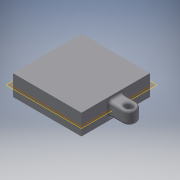
# Autodesk Inventor part: Casing_Part3
Saved by Autodesk Inventor 2019 (Build 230136000, 136)
## iProperties
Created: 2020-12-20
Part Number: Casing_Part3
Material: Generic
Document SubType Name: Modeling
Designer: nicolas
Density: 1 g/cm^3
Appearance: Default
Author: nicolas
Autodesk Inventor part; units mm, degrees
ref_plane "YZ Plane" through (0, 0, 0) normal (1, 0, 0) x (0, 1, 0)
ref_plane "XZ Plane" through (0, 0, 0) normal (0, 1, 0) x (-1, 0, 0)
ref_plane "XY Plane" through (0, 0, 0) normal (0, 0, 1) x (1, 0, 0)
sketch "Sketch1" plane through (0, 0, 0) normal (0, 1, 0) x (-1, 0, 0)
  line L0 (0, 0) -> (-50, 0)
  line L1 (-50, 0) -> (-50, -50)
  line L2 (-50, -50) -> (0, -50)
  line L3 (0, -50) -> (0, 0)
  dimension "d0" = 50
  dimension "d1" = 50
  constraints: 8 end point, 2 parallel, 1 horizontal, 1 perpendicular
  measures "d0" distance of L2.end L1.end
  measures "d1" distance of L1.end L0.end
extrude "Extrusion1" add sketch "Sketch1" along normal blind 15
ref_plane "Work Plane1" through (0, 7.5, 0) normal (0, 1, 0) x (1, 0, 0)
sketch "Sketch2" plane through (0, 7.5, 0) normal (0, 1, 0) x (1, 0, 0)
  line L0 (50, 20) -> (60, 20)
  line L1 (60, 20) -> (60, 30) construction
  line L2 (60, 30) -> (50, 30)
  line L3 (50, 30) -> (50, 20)
  line L4 (50, 20) -> (60, 30) construction
  line L5 (60, 20) -> (50, 30) construction
  line L6 (50, 0) -> (50, 50) projected
  arc A0 (60, 20) -> (60, 30) centre (60, 25) ccw
  line L7 (50, 25) -> (60, 25) construction
  point P0 (0, 0)
  dimension "d4" = 10
  dimension "d5" = 10
  constraints: 14 end point, 3 midpoint, 2 horizontal, 2 parallel, 2 point on circle, 1 centre point, 1 perpendicular
  measures "d4" distance of L1.end L2.end
  measures "d5" distance of L0.end L1.end
extrude "Extrusion2" add sketch "Sketch2" along normal mid plane 10
sketch "Sketch3" plane through (0, 12.5, 0) normal (0, 1, 0) x (1, 0, 0)
  arc A0 (60, 20) -> (60, 30) centre (60, 25) ccw projected
  point P0 (0, 0)
hole "Hole1" at (60, 12.5, -25) direction (0, -1, 0) diameter 5.5 end through all clearance for "Countersunk Flat Head Screw ISO 2009/7046" size "M5" standard "ISO"
fillet "Fillet1" radius 2 12 edges at (55, 2.5, -20) (55, 2.5, -30) (65, 2.5, -25) (55, 12.5, -30) (55, 12.5, -20) (65, 12.5, -25) (60, 12.5, -27.75) (60, 2.5, -27.75) (50, 12.5, -25) (50, 7.5, -20) (50, 2.5, -25) (50, 7.5, -30)
body "Solid1"
